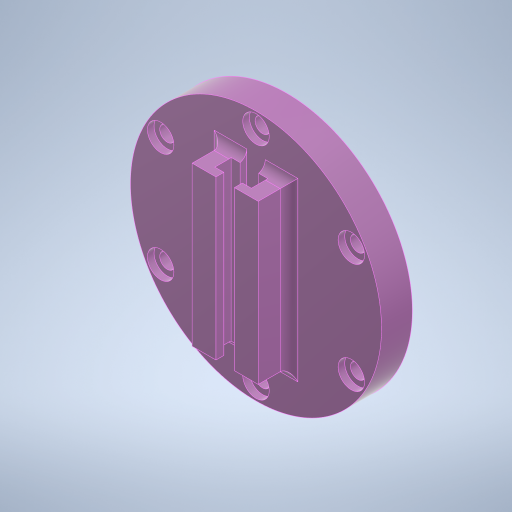
# Autodesk Inventor part: piper-GIM3505-8
Saved by Autodesk Inventor 2024 (Build 280153000, 153)
## iProperties
Created: 2025-04-03
Part Number: piper-GIM3505-8
Material: ABS プラスチック
Document SubType Name: Modeling
Designer: 1412z
Density: 1.06 g/cm^3
Appearance: 滑らか - 紫
Author: 1412z
Autodesk Inventor part; units mm, degrees
ref_plane "YZ Plane" through (0, 0, 0) normal (1, 0, 0) x (0, 1, 0)
ref_plane "XZ Plane" through (0, 0, 0) normal (0, 1, 0) x (-1, 0, 0)
ref_plane "XY Plane" through (0, 0, 0) normal (0, 0, 1) x (1, 0, 0)
sketch "スケッチ1" plane through (0, 0, 0) normal (0, 0, 1) x (1, 0, 0)
  circle A0 centre (0, 0) radius 28.5
  circle A1 centre (0, 0) radius 20
  dimension "d0" = 57
  dimension "d1" = 40
  constraints: 2 centre point, 2 coincident
  measures "d0" diameter of A0
  measures "d1" diameter of A1
extrude "押し出し1" add sketch "スケッチ1" along normal blind 10 contours A0 | A1
sketch "スケッチ2" plane through (0, 0, 0) normal (0, 0, -1) x (-1, 0, 0)
  circle A0 centre (0, 0) radius 22.5
  dimension "d4" = 45
  constraints: 1 centre point, 1 coincident
  measures "d4" diameter of A0
extrude "押し出し2" cut sketch "スケッチ2" against normal blind 5
sketch "スケッチ4" plane through (0, 0, 10) normal (0, 0, 1) x (1, 0, 0)
  circle A0 centre (0, 0) radius 25
  circle A1 centre (0, -25) radius 1.7
  circle A2 centre (21.6506, -12.5) radius 1.7
  circle A3 centre (21.6506, 12.5) radius 1.7
  circle A4 centre (0, 25) radius 1.7
  circle A5 centre (-21.6506, 12.5) radius 1.7
  circle A6 centre (-21.6506, -12.5) radius 1.7
  dimension "d15" = 50
  dimension "d16" = 3.4
  dimension "d19" = 360
  constraints: 6 centre point, 1 coincident, 1 vertical alignment, 15 other
  measures "d16" diameter of A1
extrude "押し出し4" cut sketch "スケッチ4" against normal blind 10 contours A3 A0 | A0 A3 | A2 A0 | A0 A2 | A4 A0 | A0 A4 | A1 A0 | A0 A1 | A5 A0 | A0 A5 | A6 A0 | A0 A6
sketch "スケッチ5" plane through (0, 0, 10) normal (0, 0, 1) x (1, 0, 0)
  circle A0 centre (0, 0) radius 28.5
  constraints: 1 centre point, 1 coincident
extrude "押し出し5" cut sketch "スケッチ5" against normal blind 3
sketch "スケッチ6" plane through (0, 0, 7) normal (0, 0, 1) x (1, 0, 0)
  circle A0 centre (0, 0) radius 21.5
  circle A1 centre (0, 25) radius 1.7 projected
  circle A2 centre (0, 25) radius 3
  circle A3 centre (-21.6506, 12.5) radius 3
  circle A4 centre (-21.6506, -12.5) radius 3
  circle A5 centre (0, -25) radius 3
  circle A6 centre (21.6506, -12.5) radius 3
  circle A7 centre (21.6506, 12.5) radius 3
  dimension "d25" = 43
  dimension "d26" = 6
  dimension "d29" = 360
  constraints: 7 centre point, 2 coincident, 13 other
  measures "d25" diameter of A0
  measures "d26" diameter of A2
extrude "押し出し6" cut sketch "スケッチ6" against normal blind 1.5 contours A1 | A2 | A3 | A4 | A5 | A6 | A7
sketch "スケッチ7" plane through (0, 0, 7) normal (0, 0, 1) x (1, 0, 0)
  line L0 (0, 0) -> (7.5, 0)
  line L1 (7.5, 0) -> (7.5, 18)
  line L2 (7.5, 18) -> (-7.5, 18)
  line L3 (-7.5, 18) -> (-7.5, -18)
  line L4 (-7.5, -18) -> (7.5, -18)
  line L5 (7.5, -18) -> (7.5, 0)
  dimension "d33" = 7.5
  dimension "d34" = 18
  dimension "d35" = 15
  dimension "d36" = 36
  constraints: 12 end point, 5 perpendicular, 1 horizontal, 1 point on line
  measures "d33" distance of L0.start L0.end
  measures "d34" distance of L0.end L1.end
  measures "d35" distance of L1.end L2.end
  measures "d36" distance of L2.end L3.end
extrude "押し出し7" add sketch "スケッチ7" along normal blind 7
sketch "スケッチ8" plane through (-7.5, 18, 7) normal (0, 1, 0) x (1, 0, 0)
  line L0 (15, 0) -> (0, 0) projected
  line L1 (7.5, 0) -> (9.6, 0)
  line L2 (9.6, 0) -> (9.6, -1.5)
  line L3 (9.6, -1.5) -> (5.4, -1.5)
  line L4 (5.4, -1.5) -> (5.4, 0)
  line L5 (7.5, 0) -> (5.4, 0)
  line L6 (7.5, -1.5) -> (11.65, -1.5)
  line L7 (11.65, -1.5) -> (11.65, -5.2)
  line L8 (11.65, -5.2) -> (3.35, -5.2)
  line L9 (3.35, -5.2) -> (3.35, -1.5)
  line L10 (3.35, -1.5) -> (7.5, -1.5)
  line L11 (7.5, -5.2) -> (9.6, -5.2)
  line L12 (9.6, -5.2) -> (9.6, -7)
  line L13 (0, -7) -> (15, -7) projected
  line L14 (9.6, -7) -> (5.4, -7)
  line L15 (5.4, -7) -> (5.4, -5.2)
  point P0 (7.5, 7)
  dimension "d39" = 2.1
  dimension "d40" = 1.5
  dimension "d41" = 4.2
  dimension "d42" = 4.15
  dimension "d43" = 3.7
  dimension "d44" = 8.3
  dimension "d45" = 2.1
  constraints: 28 end point, 10 point on line, 7 perpendicular, 3 midpoint, 1 collinear, 1 vertical
  measures "d39" distance of L1.start L1.end
  measures "d40" distance of L1.end L2.end
  measures "d41" distance of L2.end L3.end
  measures "d42" distance of L6.start L6.end
  measures "d43" distance of L6.end L7.end
  measures "d44" distance of L7.end L8.end
  measures "d45" distance of L11.start L11.end
extrude "押し出し8" cut sketch "スケッチ8" against normal blind 40
fillet "フィレット1" radius 2 6 edges at (-4.8, -18, 7) (4.8, -18, 7) (7.5, 0, 7) (-7.5, 0, 7) (-4.8, 18, 7) (4.8, 18, 7)
